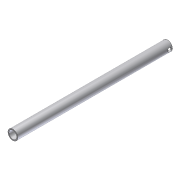
# Autodesk Inventor part: FE-00003-01
Saved by Autodesk Inventor 2012 (Build 160160000, 160)
## iProperties
Created: 2008-05-15
Part Number: FE-00003-01
Document SubType Name: Modeling
Designer: narosenberg
Density: 1 g/cm^3
Description: Rail Pin
Material: Default
Author: narosenberg
Autodesk Inventor part; units mm, degrees
ref_plane "XZ Plane" through (0, 0, 0) normal (0, 1, 0) x (-1, 0, 0)
ref_plane "XY Plane" through (0, 0, 0) normal (0, 0, 1) x (1, 0, 0)
sketch "Sketch1" plane through (0, 0, 0) normal (0, 0, 1) x (1, 0, 0)
  circle A0 centre (-10.274, 6.5449) radius 16.7005
  dimension "d0" = 33.401
  constraints: 1 centre point
  measures "d0" diameter of A0
extrude "Extrusion1" add sketch "Sketch1" along normal blind 520.7
shell "Shell1" thickness 3.3782 removed faces 2 at (-15.0414, 5.2901, 0) at (-15.0414, 5.2901, 520.7)
ref_plane "Work Plane1" through (6.4265, 6.5449, 0) normal (1, 0, 0) x (0, 1, 0)
sketch "Sketch3" plane through (6.4265, 6.5449, 0) normal (1, 0, 0) x (0, 1, 0)
  line L0 (13.3223, 0) -> (-13.3223, 0) projected
  circle A0 centre (0, 9.525) radius 6.35
  dimension "d4" = 12.7
  dimension "d5" = 9.525
  constraints: 1 centre point
  measures "d4" diameter of A0
  measures "d5" distance from line of A0.centre L0
extrude "Extrusion2" cut sketch "Sketch3" against normal through all
body "Solid1"
